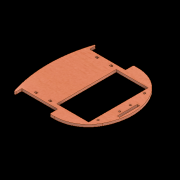
# Autodesk Inventor part: Parte inferior 2 v2
Saved by Autodesk Inventor 2022 (Build 260153000, 153)
## iProperties
Created: 2021-09-27
Part Number: Parte inferior 2 v2
Material: Madera (nogal)
Document SubType Name: Modeling
Designer: Julio R
Density: 0.55 g/cm^3
Appearance: Nogal - Natural pulido
Author: Julio R
Autodesk Inventor part; units mm, degrees
ref_plane "YZ Plane" through (0, 0, 0) normal (1, 0, 0) x (0, 1, 0)
ref_plane "XZ Plane" through (0, 0, 0) normal (0, 1, 0) x (-1, 0, 0)
ref_plane "XY Plane" through (0, 0, 0) normal (0, 0, 1) x (1, 0, 0)
sketch "Boceto2" plane through (0, 0, 0) normal (0, 1, 0) x (-1, 0, 0)
  circle A0 centre (-10.65, 0) radius 62.5
  line L0 (-63, 32.5) -> (-63, -32.5)
  line L1 (-63, -32.5) -> (-33, -32.5)
  line L2 (-33, -32.5) -> (-33, 32.5)
  line L3 (-33, 32.5) -> (-63, 32.5)
  circle A1 centre (-59.5, -29) radius 1.25
  line L4 (0, 6.809) -> (0, -6.809)
  line L5 (10.65, 0) -> (-10.65, 0) construction
  circle A2 centre (-36.5, -29) radius 1.25
  circle A3 centre (-59.5, 29) radius 1.25
  circle A4 centre (-36.5, 29) radius 1.25
  line L6 (7.5, -42.3) -> (-7.5, -42.3)
  line L7 (-7.5, -42.3) -> (-7.5, -25)
  line L8 (-7.5, -25) -> (7.5, -25)
  line L9 (7.5, -25) -> (7.5, -42.3)
  arc A5 (9, -42.3) -> (9, -33.8) centre (9, -38.05) ccw
  line L10 (9, -42.3) -> (7.5, -42.3)
  line L11 (9, -33.8) -> (7.5, -33.8)
  arc A6 (9.5, -39.2) -> (9.5, -36.9) centre (9.5, -38.05) ccw
  line L12 (9.5, -39.2) -> (7.5, -39.2)
  line L13 (7.5, -39.2) -> (7.5, -36.9)
  line L14 (7.5, -36.9) -> (9.5, -36.9)
  line L15 (9.5, -36.9) -> (9.5, -39.2)
  arc A7 (-9, -33.8) -> (-9, -42.3) centre (-9, -38.05) ccw
  line L16 (-9, -42.3) -> (-7.5, -42.3)
  line L17 (-9, -33.8) -> (-7.5, -33.8)
  arc A8 (-9.5, -36.9) -> (-9.5, -39.2) centre (-9.5, -38.05) ccw
  line L18 (-9.5, -39.2) -> (-7.5, -39.2)
  line L19 (-7.5, -39.2) -> (-7.5, -36.9)
  line L20 (-7.5, -36.9) -> (-9.5, -36.9)
  line L21 (-9.5, -36.9) -> (-9.5, -39.2)
  line L22 (7.5, 42.3) -> (-7.5, 42.3)
  line L23 (-7.5, 42.3) -> (-7.5, 25)
  line L24 (-7.5, 25) -> (7.5, 25)
  line L25 (7.5, 25) -> (7.5, 42.3)
  arc A9 (9, 33.8) -> (9, 42.3) centre (9, 38.05) ccw
  line L26 (9, 42.3) -> (7.5, 42.3)
  line L27 (9, 33.8) -> (7.5, 33.8)
  arc A10 (9.5, 36.9) -> (9.5, 39.2) centre (9.5, 38.05) ccw
  line L28 (9.5, 39.2) -> (7.5, 39.2)
  line L29 (7.5, 39.2) -> (7.5, 36.9)
  line L30 (7.5, 36.9) -> (9.5, 36.9)
  line L31 (9.5, 36.9) -> (9.5, 39.2)
  line L32 (-9, 33.8) -> (-7.5, 33.8)
  line L33 (-7.5, 36.9) -> (-9.5, 36.9)
  line L34 (-7.5, 39.2) -> (-7.5, 36.9)
  line L35 (-9.5, 36.9) -> (-9.5, 39.2)
  line L36 (-9.5, 39.2) -> (-7.5, 39.2)
  arc A11 (-9.5, 39.2) -> (-9.5, 36.9) centre (-9.5, 38.05) ccw
  line L37 (-9, 42.3) -> (-7.5, 42.3)
  arc A12 (-9, 42.3) -> (-9, 33.8) centre (-9, 38.05) ccw
  line L38 (-16, -37.25) -> (-56, -37.25)
  line L39 (-56, -37.25) -> (-56, 37.25)
  line L40 (-56, 37.25) -> (-16, 37.25)
  line L41 (-16, 37.25) -> (-16, -37.25)
  line L42 (20.3604, -4.25) -> (0.1604, -4.25)
  line L43 (0.1604, -4.25) -> (0.1604, 4.25)
  line L44 (0.1604, 4.25) -> (20.3604, 4.25)
  line L45 (20.3604, 4.25) -> (20.3604, -4.25)
  line L46 (35.3604, -42.3) -> (-56.6604, -42.3)
  line L47 (-56.6604, -42.3) -> (-56.6604, 42.3)
  line L48 (-56.6604, 42.3) -> (35.3604, 42.3)
  line L49 (35.3604, 42.3) -> (35.3604, -42.3)
  line L50 (-67, -12.5) -> (-70, -12.5)
  line L51 (-70, -12.5) -> (-70, 12.5)
  line L52 (-70, 12.5) -> (-67, 12.5)
  line L53 (-67, 12.5) -> (-67, -12.5)
  line L54 (-19.3, -12.5) -> (-32, -12.5) construction
  line L55 (-32, -12.5) -> (-32, 7.82) construction
  line L56 (-32, 7.82) -> (-19.3, 7.82) construction
  line L57 (-19.3, 7.82) -> (-19.3, -12.5) construction
  line L58 (22.5, 52.3) -> (-22.5, 52.3)
  line L59 (-22.5, 52.3) -> (-22.5, 42.3)
  line L60 (-22.5, 42.3) -> (22.5, 42.3)
  line L61 (22.5, 42.3) -> (22.5, 52.3)
  line L62 (22.5, -52.3) -> (-22.5, -52.3)
  line L63 (-22.5, -52.3) -> (-22.5, -42.3)
  line L64 (-22.5, -42.3) -> (22.5, -42.3)
  line L65 (22.5, -42.3) -> (22.5, -52.3)
  line L66 (22.5, 52.3) -> (23.5693, 52.3)
  line L67 (-22.5, 52.3) -> (-44.8693, 52.3)
  line L68 (22.5, -52.3) -> (23.5693, -52.3)
  line L69 (-22.5, -52.3) -> (-44.8693, -52.3)
  circle A13 centre (-63.6, 6.2537) radius 1.15
  circle A14 centre (-63.6, -7.2083) radius 1.15
  arc A15 (23.5693, -52.3) -> (23.5693, 52.3) centre (-127.6415, 0) ccw
  point P0 (0, 0)
  point P1 (-33, 0)
  point P2 (0, 0)
  point P3 (13.25, -38.05)
  point P4 (10.65, -38.05)
  point P5 (-13.25, -38.05)
  point P6 (-10.65, -38.05)
  point P7 (13.25, 38.05)
  point P8 (10.65, 38.05)
  point P9 (-10.65, 38.05)
  point P10 (-13.25, 38.05)
  point P11 (-16, 0)
  point P12 (20.3604, 0)
  point P13 (-67, 0)
  point P14 (-56.6604, -42.3)
  point P15 (9, 42.3)
  point P16 (47.2734, 42.3)
  point P17 (0, 52.3)
  point P18 (-22.5, -42.3)
  point P19 (22.5, -42.3)
  point P20 (22.5, 42.3)
  dimension "d128" = 125
  dimension "d52" = 65
  dimension "d53" = 30
  dimension "d56" = 3.5
  dimension "d57" = 3.5
  dimension "d60" = 23
  dimension "d63" = 58
  dimension "d78" = 15
  dimension "d79" = 17.3
  dimension "d80" = 8.5
  dimension "d81" = 1.5
  dimension "d82" = 4.25
  dimension "d83" = 1.15
  dimension "d84" = 2.3
  dimension "d86" = 2
  dimension "d87" = 25
  dimension "d88" = 7.5
  dimension "d89" = 40
  dimension "d90" = 74.5
  dimension "d91" = 16
  dimension "d92" = 20.2
  dimension "d93" = 8.5
  dimension "d94" = 3
  dimension "d95" = 25
  dimension "d98" = 11
  dimension "d99" = 12.7
  dimension "d100" = 20.32
  dimension "d101" = 1
  dimension "d102" = 20
  dimension "d108" = 10
  dimension "d113" = 45
  dimension "d114" = 13.462
  dimension "d115" = 3.4
  dimension "d116" = 2.3
  dimension "d119" = 2.3
  dimension "d120" = 33
  dimension "d122" = 160
  dimension "d127" = 15
  dimension "d133" = 10.65
  constraints: 140 end point, 41 symmetric about line, 20 point on circle, 19 parallel, 15 centre point, 12 horizontal, 9 perpendicular, 7 midpoint, 5 horizontal alignment, 4 coincident, 4 collinear, 4 point on line, 3 vertical alignment, 2 vertical, 21 other
  measures "d52" distance of L2.end L1.end
  measures "d53" distance of L1.end L0.end
  measures "d56" horizontal distance of A1.centre L0.end
  measures "d57" horizontal distance of L0.end A1.centre
  measures "d60" distance of A1.centre A2.centre
  measures "d63" distance of A1.centre A3.centre
  measures "d78" distance of L7.end L8.end
  measures "d79" distance of L6.end L7.end
  measures "d80" distance between parallel lines of L11 L10
  measures "d81" distance from line of L9 A5.centre
  measures "d82" radius of A5
  measures "d83" radius of A6
  measures "d84" distance between parallel lines of L14 L12
  measures "d86" distance from line of L13 A6.centre
  measures "d87" distance from line of point (0, 0) L8
  measures "d88" distance from line of point (0, 0) L9
  measures "d89" distance of L39.end L40.end
  measures "d90" distance of L38.end L39.end
  measures "d91" distance from line of point (0, 0) L41
  measures "d92" distance of L43.end L44.end
  measures "d93" distance of L42.end L43.end
  measures "d94" distance between parallel lines of L51 L53
  measures "d95" distance between parallel lines of L52 L50
  measures "d98" distance between parallel lines of L39 L53
  measures "d99" distance of L55.end L56.end
  measures "d100" distance of L54.end L55.end
  measures "d101" distance between parallel lines of L2 L55
  measures "d102" distance between parallel lines of L1 L54
  measures "d108" distance of L59.end L58.end
  measures "d113" distance between parallel lines of L59 L61
  measures "d114" distance of A14.centre A13.centre
  measures "d115" distance from line of L53 A13.centre
  measures "d116" diameter of A13
  measures "d119" diameter of A14
  measures "d120" distance from line of L2 point (0, 0)
  measures "d122" radius of A15
  measures "d127" distance between parallel lines of L49 L45
  measures "d133" distance of point (0, 0) point (-10.65, 0)
extrude "Extrusión4" add sketch "Boceto2" along normal blind 3 contours A0 L49 | L48 A15 A0 | L49 L46 A15 L48 | A0 A15 L46 | L66 L58 L67 A0 | A15 L48 L61 L66 | A15 L46 A5 L11 L9 L8 L7 L17 A7 L47 L1 L39 L38 L41 L40 L3 L48 A12 L32 L23 L24 L25 L27 A9 | A0 L69 L62 L68 | L68 L65 L46 A15 | L67 L59 L48 A0 | L61 L48 L26 L22 L37 L59 L58 | A0 L46 L63 L69 | L62 L63 L46 L16 L6 L10 L65 | L47 L3 L0 A13 A14 L1 A0 | A9 L27 L25 L30 A10 L28 L26 | L10 L9 L12 A6 L14 L11 A5 | L47 L1 L0 A14 A13 L3 | L3 L39 L1 L47 | L25 L24 L23 L22 | L6 L7 L8 L9 | L39 L40 L41 L38 L1 L2 L3 | L3 L2 L1 L39 | L37 L23 L36 A11 L33 L32 A12 | L28 L31 L30 L25 | A7 L17 L7 L20 A8 L18 L16 | L9 L14 L15 L12 | A13 L0 | L0 A13 | L23 L33 L35 L36 | A10 L31 | A14 L0 | L0 A14 | L18 L21 L20 L7 | L15 A6 | L35 A11 | A8 L21 | A1 | A2 | A3 | A4 | L42 L43 L44 L45 | L50 L51 L52 L53
extrude "Extrusión9" cut sketch "Boceto2" along normal blind 3 contours A0 L49 | L48 A15 A0 | L49 L46 A15 L48 | A0 A15 L46 | L66 L58 L67 A0 | A0 L69 L62 L68 | L61 L48 L26 L22 L37 L59 L58 | L62 L63 L46 L16 L6 L10 L65 | L39 L40 L41 L38 L1 L2 L3 | L3 L2 L1 L39 | L28 L31 L30 L25 | L9 L14 L15 L12 | A13 L0 | L0 A13 | L23 L33 L35 L36 | A10 L31 | A14 L0 | L0 A14 | L18 L21 L20 L7 | L15 A6 | L35 A11 | A8 L21 | A1 | A2 | A3 | A4 | L50 L51 L52 L53
fillet "Empalme6" radius 1 10 edges at (-23.5693, 1.5, 52.3) (-22.5, 1.5, 52.3) (-23.5693, 1.5, -52.3) (-22.5, 1.5, -52.3) (22.5, 1.5, -52.3) (22.5, 1.5, 52.3) (22.5, 1.5, -42.3) (-22.5, 1.5, -42.3) (-22.5, 1.5, 42.3) (22.5, 1.5, 42.3)
fillet "Empalme7" radius 43 2 edges at (44.8693, 1.5, 52.3) (44.8693, 1.5, -52.3)
